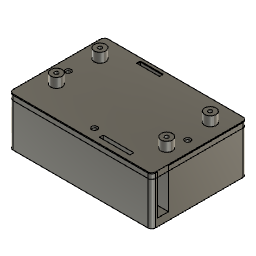
SensorEnclosure (Autodesk Fusion 360 design; units mm, degrees)
Autodesk Fusion 360 part; units mm, degrees
sketch "Sketch3" plane through (0, 0, 0) normal (0, 0, 1) x (1, 0, 0) in component "Body"
  line L0 (0, 0) -> (75, 0)
  line L1 (75, 0) -> (75, 50)
  line L2 (75, 50) -> (0, 50)
  line L3 (0, 50) -> (0, 0)
  dimension "d8" = 75
  dimension "d9" = 50
  constraint horizontal L0
  constraint vertical L1
  constraint horizontal L2
  constraint vertical L3
  constraint coincident L0.start L3.end
  measures "d8" distance of L0.start L0.end
  measures "d9" distance of L0.start L2.end
extrude "Extrude1" add sketch "Sketch3" along normal blind 25 makes body 1 in component "Body"
fillet "Fillet1" radius 2 4 edges at (0, 0, 12.5) (75, 0, 12.5) (75, 50, 12.5) (0, 50, 12.5) on bodies 1 in component "Body"
extrude "Extrude1'" add 1 faces at (49.3333, 16.6667, 25) along direction (0, 0, 1) blind 3 separate body on bodies 1 makes body 2 in component "Top"
sketch "Sketch6" plane through (0, 0, 25) normal (0, 0, 1) x (-1, 0, 0) in component "Body"
  arc A0 (-2, -50) -> (0, -48) centre (-2, -48) ccw
  line L0 (0, -48) -> (0, -2)
  arc A1 (0, -2) -> (-2, 0) centre (-2, -2) ccw
  line L1 (-2, 0) -> (-73, 0)
  arc A2 (-73, 0) -> (-75, -2) centre (-73, -2) ccw
  line L2 (-75, -2) -> (-75, -48)
  arc A3 (-75, -48) -> (-73, -50) centre (-73, -48) ccw
  line L3 (-73, -50) -> (-2, -50)
  line L4 (-12.6, -47) -> (-62.8, -47)
  line L5 (-62.8, -47) -> (-62.8, -8.8)
  line L6 (-62.8, -8.8) -> (-12.6, -8.8)
  line L7 (-12.6, -8.8) -> (-12.6, -47)
  dimension "d19" = 50.2
  dimension "d20" = 38.2
  constraint horizontal L4
  constraint vertical L5
  constraint horizontal L6
  constraint vertical L7
  measures "d19" distance of L4.start L4.end
  measures "d20" distance of L4.start L6.end
extrude "Extrude2" cut sketch "Sketch6" against normal blind 21 contours L4 L5 L6 L7 bodies 1 in component "Body"
sketch "Sketch8" plane through (0, 0, 25) normal (0, 0, 1) x (-1, 0, 0) in component "Body"
  line L0 (-62.8, -47) -> (-62.8, -8.8)
  line L1 (-62.8, -8.8) -> (-12.6, -8.8)
  line L2 (-12.6, -8.8) -> (-12.6, -47)
  line L3 (-12.6, -47) -> (-62.8, -47)
  arc A0 (-2, -50) -> (0, -48) centre (-2, -48) ccw
  line L4 (0, -48) -> (0, -2)
  arc A1 (0, -2) -> (-2, 0) centre (-2, -2) ccw
  line L5 (-2, 0) -> (-73, 0)
  arc A2 (-73, 0) -> (-75, -2) centre (-73, -2) ccw
  line L6 (-75, -2) -> (-75, -48)
  arc A3 (-75, -48) -> (-73, -50) centre (-73, -48) ccw
  line L7 (-73, -50) -> (-2, -50)
  line L8 (-42.5, -3) -> (-75, -3)
  line L9 (-75, -3) -> (-75, -8.8)
  line L10 (-75, -8.8) -> (-42.5, -8.8)
  line L11 (-42.5, -8.8) -> (-42.5, -3)
  line L12 (-35.5, -3) -> (0, -3)
  line L13 (0, -3) -> (0, -8.8)
  line L14 (0, -8.8) -> (-35.5, -8.8)
  line L15 (-35.5, -8.8) -> (-35.5, -3)
  constraint horizontal L8
  constraint vertical L9
  constraint horizontal L10
  constraint vertical L11
  constraint coincident L6 L9.end
  constraint horizontal L12
  constraint vertical L13
  constraint horizontal L14
  constraint vertical L15
  constraint coincident L4 L13.end
extrude "Extrude3" cut sketch "Sketch8" against normal blind 21 contours L1 L6 L8 L9 L10 L11 | L1 L4 L12 L13 L14 L15 bodies 1 in component "Body"
sketch "Sketch9" plane through (0, 47, 0) normal (0, -1, 0) x (1, 0, 0) in component "Body"
  line L0 (62.8, 25) -> (12.6, 25)
  line L1 (12.6, 25) -> (12.6, 4)
  line L2 (12.6, 4) -> (62.8, 4)
  line L3 (62.8, 4) -> (62.8, 25)
  line L4 (20.5169, 25) -> (32.5169, 25)
  line L5 (32.5169, 25) -> (32.5169, 13)
  line L6 (32.5169, 13) -> (20.5169, 13)
  line L7 (20.5169, 13) -> (20.5169, 25)
  dimension "d31" = 12
  dimension "d32" = 12
  constraint horizontal L4
  constraint vertical L5
  constraint horizontal L6
  constraint vertical L7
  constraint coincident L0 L4.start
  measures "d31" distance of L4.start L4.end
  measures "d32" distance of L4.start L6.end
extrude "Extrude4" cut sketch "Sketch9" against normal blind 1.5 contours L0 L4 L5 L6 L7 bodies 1 in component "Body"
sketch "Sketch10" plane through (0, 0, 25) normal (0, 0, 1) x (-1, 0, 0) in component "Body"
  line L0 (-20.5169, -47) -> (-20.5169, -48.5)
  line L1 (-20.5169, -48.5) -> (-32.5169, -48.5)
  line L2 (-32.5169, -48.5) -> (-32.5169, -47)
  line L3 (-32.5169, -47) -> (-62.8, -47)
  line L4 (-62.8, -47) -> (-62.8, -8.8)
  line L5 (-62.8, -8.8) -> (-75, -8.8)
  line L6 (-75, -8.8) -> (-75, -48)
  arc A0 (-75, -48) -> (-73, -50) centre (-73, -48) ccw
  line L7 (-73, -50) -> (-2, -50)
  arc A1 (-2, -50) -> (0, -48) centre (-2, -48) ccw
  line L8 (0, -48) -> (0, -8.8)
  line L9 (0, -8.8) -> (-12.6, -8.8)
  line L10 (-12.6, -8.8) -> (-12.6, -47)
  line L11 (-12.6, -47) -> (-20.5169, -47)
  line L12 (-3, -47) -> (-9.589, -47)
  line L13 (-9.589, -47) -> (-9.589, -28.4)
  line L14 (-9.589, -28.4) -> (-3, -28.4)
  line L15 (-3, -28.4) -> (-3, -47)
  line L16 (-3, -21.4819) -> (-9.589, -21.4819)
  line L17 (-9.589, -21.4819) -> (-9.589, -11.7871)
  line L18 (-9.589, -11.7871) -> (-3, -11.7871)
  line L19 (-3, -11.7871) -> (-3, -21.4819)
  constraint horizontal L12
  constraint vertical L13
  constraint horizontal L14
  constraint vertical L15
  constraint horizontal L16
  constraint vertical L17
  constraint horizontal L18
  constraint vertical L19
extrude "Extrude5" cut sketch "Sketch10" against normal blind 20.9 contours L12 L13 L14 L15 | L16 L17 L18 L19 bodies 1 in component "Body"
sketch "Sketch11" plane through (0, 0, 25) normal (0, 0, 1) x (-1, 0, 0) in component "Body"
  line L0 (-9.589, -21.4819) -> (-9.589, -11.7871)
  line L1 (-9.589, -11.7871) -> (-3, -11.7871)
  line L2 (-3, -11.7871) -> (-3, -21.4819)
  line L3 (-3, -21.4819) -> (-9.589, -21.4819)
  line L4 (-9.589, -47) -> (-9.589, -28.4)
  line L5 (-9.589, -28.4) -> (-3, -28.4)
  line L6 (-3, -28.4) -> (-3, -47)
  line L7 (-3, -47) -> (-9.589, -47)
  line L8 (-20.5169, -47) -> (-20.5169, -48.5)
  line L9 (-20.5169, -48.5) -> (-32.5169, -48.5)
  line L10 (-32.5169, -48.5) -> (-32.5169, -47)
  line L11 (-32.5169, -47) -> (-62.8, -47)
  line L12 (-62.8, -47) -> (-62.8, -8.8)
  line L13 (-62.8, -8.8) -> (-75, -8.8)
  line L14 (-75, -8.8) -> (-75, -48)
  arc A0 (-75, -48) -> (-73, -50) centre (-73, -48) ccw
  line L15 (-73, -50) -> (-2, -50)
  arc A1 (-2, -50) -> (0, -48) centre (-2, -48) ccw
  line L16 (0, -48) -> (0, -8.8)
  line L17 (0, -8.8) -> (-12.6, -8.8)
  line L18 (-12.6, -8.8) -> (-12.6, -47)
  line L19 (-12.6, -47) -> (-20.5169, -47)
  line L20 (-71.9773, -11.7761) -> (-65.7622, -11.7761)
  line L21 (-65.7622, -11.7761) -> (-65.7622, -21.4143)
  line L22 (-65.7622, -21.4143) -> (-71.9773, -21.4143)
  line L23 (-71.9773, -21.4143) -> (-71.9773, -11.7761)
  line L24 (-65.7622, -47.0153) -> (-71.9773, -47.0153)
  line L25 (-71.9773, -47.0153) -> (-71.9773, -28.4)
  line L26 (-71.9773, -28.4) -> (-65.7622, -28.4)
  line L27 (-65.7622, -28.4) -> (-65.7622, -47.0153)
  constraint horizontal L20
  constraint vertical L21
  constraint horizontal L22
  constraint vertical L23
  constraint horizontal L24
  constraint vertical L25
  constraint horizontal L26
  constraint vertical L27
extrude "Extrude6" cut sketch "Sketch11" against normal blind 20.9 contours L20 L21 L22 L23 | L24 L25 L26 L27 bodies 1 in component "Body"
sketch "Sketch1" plane through (0, 0, 28) normal (0, 0, 1) x (-1, 0, 0) in component "Top"
  arc A0 (-2, -50) -> (0, -48) centre (-2, -48) ccw
  line L0 (0, -48) -> (0, -2)
  arc A1 (0, -2) -> (-2, 0) centre (-2, -2) ccw
  line L1 (-2, 0) -> (-73, 0)
  arc A2 (-73, 0) -> (-75, -2) centre (-73, -2) ccw
  line L2 (-75, -2) -> (-75, -48)
  arc A3 (-75, -48) -> (-73, -50) centre (-73, -48) ccw
  line L3 (-73, -50) -> (-2, -50)
  line L4 (-20.5, -48.5) -> (-32.5, -48.5)
  line L5 (-32.5, -48.5) -> (-32.5, -46.5)
  line L6 (-32.5, -46.5) -> (-20.5, -46.5)
  line L7 (-20.5, -46.5) -> (-20.5, -48.5)
  dimension "d54" = 2
  constraint horizontal L4
  constraint vertical L5
  constraint horizontal L6
  constraint vertical L7
  measures "d54" distance of L4.start L6.end
sketch "Sketch3 (2)" plane through (0, 0, 28) normal (0, 0, 1) x (-1, 0, 0) in component "Top"
  arc A0 (-2, -50) -> (0, -48) centre (-2, -48) ccw
  line L0 (0, -48) -> (0, -2)
  arc A1 (0, -2) -> (-2, 0) centre (-2, -2) ccw
  line L1 (-2, 0) -> (-73, 0)
  arc A2 (-73, 0) -> (-75, -2) centre (-73, -2) ccw
  line L2 (-75, -2) -> (-75, -48)
  arc A3 (-75, -48) -> (-73, -50) centre (-73, -48) ccw
  line L3 (-73, -50) -> (-2, -50)
  circle A4 centre (-8.7934, -38.9524) radius 3
  circle A5 centre (-8.7934, -16.0408) radius 3
  circle A6 centre (-66.785, -39.0237) radius 3
  circle A7 centre (-66.8877, -15.9333) radius 3
  dimension "d59" = 6
  dimension "d60" = 6
  dimension "d61" = 6
  dimension "d62" = 6
  measures "d59" diameter of A4
  measures "d60" diameter of A5
  measures "d61" diameter of A6
  measures "d62" diameter of A7
extrude "Extrude3'" add sketch "Sketch3 (2)" along normal blind 5 contours A4 | A5 | A6 | A7 bodies 2 in component "Top"
sketch "Sketch4" plane through (0, 0, 33) normal (0, 0, 1) x (-1, 0, 0) in component "Top"
  circle A0 centre (-8.7934, -38.9524) radius 3
  circle A1 centre (-8.7934, -38.9524) radius 1
  circle A2 centre (-66.7401, -38.996) radius 1
  dimension "d65" = 2
  dimension "d66" = 2
  constraint concentric A0 A1
  measures "d65" diameter of A1
  measures "d66" diameter of A2
sketch "Sketch5" plane through (0, 0, 33) normal (0, 0, 1) x (-1, 0, 0) in component "Top"
  circle A0 centre (-8.7934, -16.0408) radius 3
  circle A1 centre (-8.7934, -16.0408) radius 1
  circle A2 centre (-66.9224, -15.9095) radius 1
  dimension "d67" = 2
  dimension "d68" = 2
  constraint concentric A0 A1
  measures "d67" diameter of A1
  measures "d68" diameter of A2
extrude "Extrude4'" cut sketch "Sketch4" sketch "Sketch5" against normal blind 5 contours A1 | A2 of sketch 2 contours A1 | A2 bodies 2 in component "Top"
ref_plane "WorkPlane1" through (3.0798, -18.8013, 2.7227) normal (-1, 0, 0) x (0, 1, 0)
sketch "Sketch5 (2)" plane through (0, 0, 13.2227) normal (0, 0, 1) x (-1, 0, 0)
  line L0 (-39.0798, 21.7013) -> (-6.5798, 21.7013)
  line L1 (-6.5798, 21.7013) -> (-6.5798, 15.9014)
  line L2 (-6.5798, 15.9014) -> (0.4202, 15.9014)
  line L3 (0.4202, 15.9014) -> (0.4202, 21.7013)
  line L4 (0.4202, 21.7013) -> (35.9202, 21.7013)
  line L5 (35.9202, 21.7013) -> (35.9202, 22.7013)
  arc A0 (35.9202, 22.7013) -> (33.9202, 24.7013) centre (33.9202, 22.7013) ccw
  line L6 (33.9202, 24.7013) -> (-37.0798, 24.7013)
  arc A1 (-37.0798, 24.7013) -> (-39.0798, 22.7013) centre (-37.0798, 22.7013) ccw
  line L7 (-39.0798, 22.7013) -> (-39.0798, 21.7013)
  circle A2 centre (-3.0194, 18.172) radius 1
  dimension "d75" = 2
  measures "d75" diameter of A2
sketch "Sketch6 (2)" plane through (0, 0, 13.2227) normal (0, 0, 1) x (-1, 0, 0)
  line L0 (15.4033, -23.7986) -> (3.4033, -23.7986)
  line L1 (3.4033, -23.7986) -> (3.4033, -22.2986)
  line L2 (3.4033, -22.2986) -> (-26.8798, -22.2986)
  line L3 (-26.8798, -22.2986) -> (-26.8798, 15.9014)
  line L4 (-26.8798, 15.9014) -> (-39.0798, 15.9014)
  line L5 (-39.0798, 15.9014) -> (-39.0798, -23.2987)
  arc A0 (-39.0798, -23.2987) -> (-37.0798, -25.2987) centre (-37.0798, -23.2987) ccw
  line L6 (-37.0798, -25.2987) -> (33.9202, -25.2987)
  arc A1 (33.9202, -25.2987) -> (35.9202, -23.2987) centre (33.9202, -23.2987) ccw
  line L7 (35.9202, -23.2987) -> (35.9202, 15.9014)
  line L8 (35.9202, 15.9014) -> (23.3202, 15.9014)
  line L9 (23.3202, 15.9014) -> (23.3202, -22.2986)
  line L10 (23.3202, -22.2986) -> (15.4033, -22.2986)
  line L11 (26.3312, -22.2987) -> (26.3312, -3.6986)
  line L12 (26.3312, -3.6986) -> (32.9202, -3.6986)
  line L13 (32.9202, -3.6986) -> (32.9202, -22.2987)
  line L14 (32.9202, -22.2987) -> (26.3312, -22.2987)
  line L15 (26.3312, 3.2194) -> (26.3312, 12.9142)
  line L16 (26.3312, 12.9142) -> (32.9202, 12.9142)
  line L17 (32.9202, 12.9142) -> (32.9202, 3.2194)
  line L18 (32.9202, 3.2194) -> (26.3312, 3.2194)
  line L19 (-29.8421, 12.9253) -> (-29.8421, 3.287)
  line L20 (-29.8421, 3.287) -> (-36.0572, 3.287)
  line L21 (-36.0572, 3.287) -> (-36.0572, 12.9253)
  line L22 (-36.0572, 12.9253) -> (-29.8421, 12.9253)
  line L23 (-36.0572, -22.314) -> (-36.0572, -3.6986)
  line L24 (-36.0572, -3.6986) -> (-29.8421, -3.6986)
  line L25 (-29.8421, -3.6986) -> (-29.8421, -22.314)
  line L26 (-29.8421, -22.314) -> (-36.0572, -22.314)
  circle A2 centre (29.7902, -0.2383) radius 1
  circle A3 centre (-32.9496, -0.2383) radius 1
  line L27 (15.4033, -22.2986) -> (15.4033, -23.7986)
  dimension "d78" = 2
  dimension "d79" = 2
  measures "d78" diameter of A2
  measures "d79" diameter of A3
sketch "Sketch15" plane through (0, 0, 25) normal (0, 0, 1) x (-1, 0, 0) in component "Body"
  line L0 (-71.9773, -47.0153) -> (-71.9773, -28.4)
  line L1 (-71.9773, -28.4) -> (-65.7622, -28.4)
  line L2 (-65.7622, -28.4) -> (-65.7622, -47.0153)
  line L3 (-65.7622, -47.0153) -> (-71.9773, -47.0153)
  line L4 (-65.7622, -11.7761) -> (-65.7622, -21.4143)
  line L5 (-65.7622, -21.4143) -> (-71.9773, -21.4143)
  line L6 (-71.9773, -21.4143) -> (-71.9773, -11.7761)
  line L7 (-71.9773, -11.7761) -> (-65.7622, -11.7761)
  line L8 (-9.589, -21.4819) -> (-9.589, -11.7871)
  line L9 (-9.589, -11.7871) -> (-3, -11.7871)
  line L10 (-3, -11.7871) -> (-3, -21.4819)
  line L11 (-3, -21.4819) -> (-9.589, -21.4819)
  line L12 (-9.589, -47) -> (-9.589, -28.4)
  line L13 (-9.589, -28.4) -> (-3, -28.4)
  line L14 (-3, -28.4) -> (-3, -47)
  line L15 (-3, -47) -> (-9.589, -47)
  line L16 (-20.5169, -47) -> (-20.5169, -48.5)
  line L17 (-20.5169, -48.5) -> (-32.5169, -48.5)
  line L18 (-32.5169, -48.5) -> (-32.5169, -47)
  line L19 (-32.5169, -47) -> (-62.8, -47)
  line L20 (-62.8, -47) -> (-62.8, -8.8)
  line L21 (-62.8, -8.8) -> (-75, -8.8)
  line L22 (-75, -8.8) -> (-75, -48)
  arc A0 (-75, -48) -> (-73, -50) centre (-73, -48) ccw
  line L23 (-73, -50) -> (-2, -50)
  arc A1 (-2, -50) -> (0, -48) centre (-2, -48) ccw
  line L24 (0, -48) -> (0, -8.8)
  line L25 (0, -8.8) -> (-12.6, -8.8)
  line L26 (-12.6, -8.8) -> (-12.6, -47)
  line L27 (-12.6, -47) -> (-20.5169, -47)
  circle A2 centre (-6.1009, -24.9964) radius 1
  dimension "d95" = 2
  measures "d95" diameter of A2
extrude "Extrude12" cut sketch "Sketch15" against normal blind 6 contours A2 bodies 1 in component "Body"
sketch "Sketch16" plane through (0, 0, 25) normal (0, 0, 1) x (-1, 0, 0) in component "Body"
  circle A0 centre (-6.1009, -24.9964) radius 1
  line L0 (-71.9773, -47.0153) -> (-71.9773, -28.4)
  line L1 (-71.9773, -28.4) -> (-65.7622, -28.4)
  line L2 (-65.7622, -28.4) -> (-65.7622, -47.0153)
  line L3 (-65.7622, -47.0153) -> (-71.9773, -47.0153)
  line L4 (-65.7622, -11.7761) -> (-65.7622, -21.4143)
  line L5 (-65.7622, -21.4143) -> (-71.9773, -21.4143)
  line L6 (-71.9773, -21.4143) -> (-71.9773, -11.7761)
  line L7 (-71.9773, -11.7761) -> (-65.7622, -11.7761)
  line L8 (-9.589, -21.4819) -> (-9.589, -11.7871)
  line L9 (-9.589, -11.7871) -> (-3, -11.7871)
  line L10 (-3, -11.7871) -> (-3, -21.4819)
  line L11 (-3, -21.4819) -> (-9.589, -21.4819)
  line L12 (-9.589, -47) -> (-9.589, -28.4)
  line L13 (-9.589, -28.4) -> (-3, -28.4)
  line L14 (-3, -28.4) -> (-3, -47)
  line L15 (-3, -47) -> (-9.589, -47)
  line L16 (-20.5169, -47) -> (-20.5169, -48.5)
  line L17 (-20.5169, -48.5) -> (-32.5169, -48.5)
  line L18 (-32.5169, -48.5) -> (-32.5169, -47)
  line L19 (-32.5169, -47) -> (-62.8, -47)
  line L20 (-62.8, -47) -> (-62.8, -8.8)
  line L21 (-62.8, -8.8) -> (-75, -8.8)
  line L22 (-75, -8.8) -> (-75, -48)
  arc A1 (-75, -48) -> (-73, -50) centre (-73, -48) ccw
  line L23 (-73, -50) -> (-2, -50)
  arc A2 (-2, -50) -> (0, -48) centre (-2, -48) ccw
  line L24 (0, -48) -> (0, -8.8)
  line L25 (0, -8.8) -> (-12.6, -8.8)
  line L26 (-12.6, -8.8) -> (-12.6, -47)
  line L27 (-12.6, -47) -> (-20.5169, -47)
  circle A3 centre (-68.8985, -25.0031) radius 1
  dimension "d98" = 2
  measures "d98" diameter of A3
extrude "Extrude13" cut sketch "Sketch16" against normal blind 6 contours A3 bodies 1 in component "Body"
sketch "Sketch11 (2)" plane through (0, 0, 28) normal (0, 0, 1) x (-1, 0, 0) in component "Top"
  circle A0 centre (-8.7934, -38.9524) radius 3
  circle A1 centre (-66.785, -39.0237) radius 3
  circle A2 centre (-8.7934, -16.0408) radius 3
  circle A3 centre (-66.8877, -15.9333) radius 3
  arc A4 (-2, -50) -> (0, -48) centre (-2, -48) ccw
  line L0 (0, -48) -> (0, -2)
  arc A5 (0, -2) -> (-2, 0) centre (-2, -2) ccw
  line L1 (-2, 0) -> (-73, 0)
  arc A6 (-73, 0) -> (-75, -2) centre (-73, -2) ccw
  line L2 (-75, -2) -> (-75, -48)
  arc A7 (-75, -48) -> (-73, -50) centre (-73, -48) ccw
  line L3 (-73, -50) -> (-2, -50)
  circle A8 centre (-39.003, -5.8917) radius 1.5
  dimension "d116" = 3
  measures "d116" diameter of A8
extrude "Extrude8" cut sketch "Sketch11 (2)" against normal blind 3 contours A8 bodies 2 in component "Top"
sketch "Sketch18" plane through (0, 0, 25) normal (0, 0, 1) x (-1, 0, 0) in component "Body"
  line L0 (-75, -3) -> (-42.5, -3)
  line L1 (-42.5, -3) -> (-42.5, -8.8)
  line L2 (-42.5, -8.8) -> (-35.5, -8.8)
  line L3 (-35.5, -8.8) -> (-35.5, -3)
  line L4 (-35.5, -3) -> (0, -3)
  line L5 (0, -3) -> (0, -2)
  arc A0 (0, -2) -> (-2, 0) centre (-2, -2) ccw
  line L6 (-2, 0) -> (-73, 0)
  arc A1 (-73, 0) -> (-75, -2) centre (-73, -2) ccw
  line L7 (-75, -2) -> (-75, -3)
  circle A2 centre (-39.0031, -5.8956) radius 1
  dimension "d119" = 2
  measures "d119" diameter of A2
extrude "Extrude17" cut sketch "Sketch18" against normal blind 6 contours A2 bodies 1 in component "Body"
sketch "Sketch19" plane through (0, 0, 4) normal (0, 0, 1) x (-1, 0, 0) in component "Body"
  line L0 (-62.8, -8.8) -> (-62.8, -47)
  line L1 (-62.8, -47) -> (-12.6, -47)
  line L2 (-12.6, -47) -> (-12.6, -8.8)
  line L3 (-12.6, -8.8) -> (0, -8.8)
  line L4 (0, -8.8) -> (0, -3)
  line L5 (0, -3) -> (-35.5, -3)
  line L6 (-35.5, -3) -> (-35.5, -8.8)
  line L7 (-35.5, -8.8) -> (-42.5, -8.8)
  line L8 (-42.5, -8.8) -> (-42.5, -3)
  line L9 (-42.5, -3) -> (-75, -3)
  line L10 (-75, -3) -> (-75, -8.8)
  line L11 (-75, -8.8) -> (-62.8, -8.8)
  line L12 (-42.5, -3) -> (-62.5, -3)
  line L13 (-62.5, -3) -> (-62.5, -5)
  line L14 (-62.5, -5) -> (-42.5, -5)
  line L15 (-42.5, -5) -> (-42.5, -3)
  dimension "d122" = 20
  dimension "d123" = 2
  constraint horizontal L12
  constraint vertical L13
  constraint horizontal L14
  constraint vertical L15
  constraint coincident L8.end L9.start
  measures "d122" distance of L8.end L12.end
  measures "d123" distance of L8.end L14.end
extrude "Extrude18" add sketch "Sketch19" along normal blind 7 contours L8 L9 L12 L13 L14 L15 bodies 1 in component "Body"
sketch "Sketch12" plane through (0, 0, 28) normal (0, 0, 1) x (-1, 0, 0) in component "Top"
  circle A0 centre (-39.003, -5.8917) radius 1.5
  circle A1 centre (-8.7934, -38.9524) radius 3
  circle A2 centre (-66.785, -39.0237) radius 3
  circle A3 centre (-8.7934, -16.0408) radius 3
  circle A4 centre (-66.8877, -15.9333) radius 3
  arc A5 (-2, -50) -> (0, -48) centre (-2, -48) ccw
  line L0 (0, -48) -> (0, -2)
  arc A6 (0, -2) -> (-2, 0) centre (-2, -2) ccw
  line L1 (-2, 0) -> (-73, 0)
  arc A7 (-73, 0) -> (-75, -2) centre (-73, -2) ccw
  line L2 (-75, -2) -> (-75, -48)
  arc A8 (-75, -48) -> (-73, -50) centre (-73, -48) ccw
  line L3 (-73, -50) -> (-2, -50)
  line L4 (-44.4921, -2.9973) -> (-60.4921, -2.9973)
  line L5 (-60.4921, -2.9973) -> (-60.4921, -4.9973)
  line L6 (-60.4921, -4.9973) -> (-44.4921, -4.9973)
  line L7 (-44.4921, -4.9973) -> (-44.4921, -2.9973)
  dimension "d128" = 16
  dimension "d129" = 2
  constraint horizontal L4
  constraint vertical L5
  constraint horizontal L6
  constraint vertical L7
  measures "d128" distance of L4.start L4.end
  measures "d129" distance of L4.start L6.end
extrude "Extrude9" cut sketch "Sketch12" against normal blind 3 contours L4 L5 L6 L7 bodies 2 in component "Top"
sketch "Sketch13" plane through (0, 0, 28) normal (0, 0, 1) x (-1, 0, 0) in component "Top"
  line L0 (-60.4921, -2.9973) -> (-44.4921, -2.9973)
  line L1 (-44.4921, -2.9973) -> (-44.4921, -4.9973)
  line L2 (-44.4921, -4.9973) -> (-60.4921, -4.9973)
  line L3 (-60.4921, -4.9973) -> (-60.4921, -2.9973)
  circle A0 centre (-39.003, -5.8917) radius 1.5
  circle A1 centre (-8.7934, -38.9524) radius 3
  circle A2 centre (-66.785, -39.0237) radius 3
  circle A3 centre (-8.7934, -16.0408) radius 3
  circle A4 centre (-66.8877, -15.9333) radius 3
  arc A5 (-2, -50) -> (0, -48) centre (-2, -48) ccw
  line L4 (0, -48) -> (0, -2)
  arc A6 (0, -2) -> (-2, 0) centre (-2, -2) ccw
  line L5 (-2, 0) -> (-73, 0)
  arc A7 (-73, 0) -> (-75, -2) centre (-73, -2) ccw
  line L6 (-75, -2) -> (-75, -48)
  arc A8 (-75, -48) -> (-73, -50) centre (-73, -48) ccw
  line L7 (-73, -50) -> (-2, -50)
  circle A9 centre (-6.1081, -24.9987) radius 1.5
  dimension "d132" = 3
  measures "d132" diameter of A9
extrude "Extrude10" cut sketch "Sketch13" against normal blind 3 contours A9 bodies 2 in component "Top"
sketch "Sketch14" plane through (0, 0, 28) normal (0, 0, 1) x (-1, 0, 0) in component "Top"
  circle A0 centre (-6.1081, -24.9987) radius 1.5
  line L0 (-60.4921, -2.9973) -> (-44.4921, -2.9973)
  line L1 (-44.4921, -2.9973) -> (-44.4921, -4.9973)
  line L2 (-44.4921, -4.9973) -> (-60.4921, -4.9973)
  line L3 (-60.4921, -4.9973) -> (-60.4921, -2.9973)
  circle A1 centre (-39.003, -5.8917) radius 1.5
  circle A2 centre (-8.7934, -38.9524) radius 3
  circle A3 centre (-66.785, -39.0237) radius 3
  circle A4 centre (-8.7934, -16.0408) radius 3
  circle A5 centre (-66.8877, -15.9333) radius 3
  arc A6 (-2, -50) -> (0, -48) centre (-2, -48) ccw
  line L4 (0, -48) -> (0, -2)
  arc A7 (0, -2) -> (-2, 0) centre (-2, -2) ccw
  line L5 (-2, 0) -> (-73, 0)
  arc A8 (-73, 0) -> (-75, -2) centre (-73, -2) ccw
  line L6 (-75, -2) -> (-75, -48)
  arc A9 (-75, -48) -> (-73, -50) centre (-73, -48) ccw
  line L7 (-73, -50) -> (-2, -50)
  circle A10 centre (-68.8989, -24.9991) radius 1.5
  dimension "d135" = 3
  measures "d135" diameter of A10
extrude "Extrude11" cut sketch "Sketch14" against normal blind 3 contours A10 bodies 2 in component "Top"
sketch "Sketch16 (2)" plane through (0, 0, 28) normal (0, 0, 1) x (-1, 0, 0) in component "Top"
  circle A0 centre (-68.8989, -24.9991) radius 1.5
  circle A1 centre (-6.1081, -24.9987) radius 1.5
  line L0 (-60.4921, -2.9973) -> (-44.4921, -2.9973)
  line L1 (-44.4921, -2.9973) -> (-44.4921, -4.9973)
  line L2 (-44.4921, -4.9973) -> (-60.4921, -4.9973)
  line L3 (-60.4921, -4.9973) -> (-60.4921, -2.9973)
  circle A2 centre (-39.003, -5.8917) radius 1.5
  circle A3 centre (-8.7934, -38.9524) radius 3
  circle A4 centre (-66.785, -39.0237) radius 3
  circle A5 centre (-8.7934, -16.0408) radius 3
  circle A6 centre (-66.8877, -15.9333) radius 3
  arc A7 (-2, -50) -> (0, -48) centre (-2, -48) ccw
  line L4 (0, -48) -> (0, -2)
  arc A8 (0, -2) -> (-2, 0) centre (-2, -2) ccw
  line L5 (-2, 0) -> (-73, 0)
  arc A9 (-73, 0) -> (-75, -2) centre (-73, -2) ccw
  line L6 (-75, -2) -> (-75, -48)
  arc A10 (-75, -48) -> (-73, -50) centre (-73, -48) ccw
  line L7 (-73, -50) -> (-2, -50)
  line L8 (-20.5071, -48.5022) -> (-32.5071, -48.5022)
  line L9 (-32.5071, -48.5022) -> (-32.5071, -46.5022)
  line L10 (-32.5071, -46.5022) -> (-20.5071, -46.5022)
  line L11 (-20.5071, -46.5022) -> (-20.5071, -48.5022)
  dimension "d140" = 12
  dimension "d141" = 2
  constraint horizontal L8
  constraint vertical L9
  constraint horizontal L10
  constraint vertical L11
  measures "d140" distance of L8.start L8.end
  measures "d141" distance of L8.start L10.end
extrude "Extrude19" cut sketch "Sketch16 (2)" against normal blind 3 contours L8 L9 L10 L11 sketch seen with x (1, 0, 0) y (0, 1, 0) z (0, 0, 1) at (-0.0033, 0.0502, -2.5) bodies 1 in component "Body"
extrude "Extrude12'" cut sketch "Sketch16 (2)" against normal blind 3 contours L8 L9 L10 L11 bodies 2 in component "Top"
component "Sensor Enclosure" placed x (1, 0, 0) y (0, 1, 0) z (0, 0, 1) at (0, 0, 0)
component "Body" placed x (1, 0, 0) y (0, 1, 0) z (0, 0, 1) at (-35.9202, -24.7013, -11.7773) in component "Sensor Enclosure"
component "Top" placed x (1, 0, 0) y (0, 1, 0) z (0, 0, 1) at (-35.9234, -24.6511, -14.2773) in component "Sensor Enclosure"
equation "Width = 50 mm"
equation "Length = 75 mm"
equation "Height = 25 mm"
equation "wall = 3 mm"
equation "Wsensor = 38 mm"
equation "Lsensor = 50 mm"
equation "Hsensor = 20.9 mm"
equation "d8 = Length"
equation "d9 = Width"
equation "d10 = Height"
equation "d19 = Lsensor + 0.2 mm"
equation "d20 = Wsensor + 0.2 mm"
equation "d21 = -Hsensor - 0.1 mm"
equation "d27 = -Hsensor - 0.1 mm"
equation "d41 = -Hsensor"
equation "d49 = -Hsensor"
